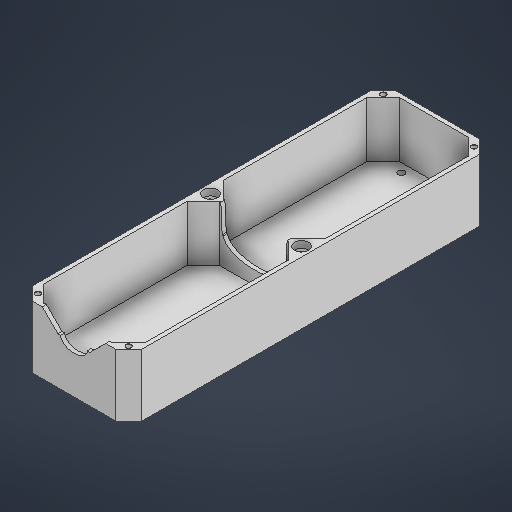
# Autodesk Inventor part: DriverFesting
Saved by Autodesk Inventor 2026.1 (Build 301233000, 233)
## iProperties
Created: 2026-01-13
Part Number: DriverFesting
Material: Generic
Document SubType Name: Modeling
Designer: Brynjar
Density: 1 g/cm^3
Appearance: Default
Author: Brynjar
Autodesk Inventor part; units mm, degrees
ref_plane "YZ Plane" through (0, 0, 0) normal (1, 0, 0) x (0, 1, 0)
ref_plane "XZ Plane" through (0, 0, 0) normal (0, 1, 0) x (-1, 0, 0)
ref_plane "XY Plane" through (0, 0, 0) normal (0, 0, 1) x (1, 0, 0)
sketch "Sketch1" plane through (0, 0, 0) normal (0, 1, 0) x (-1, 0, 0)
  line L0 (-15, -136) -> (-66, -136)
  line L1 (-78, -148) -> (-78, -254)
  line L2 (-66, -266) -> (-15, -266)
  line L3 (-3, -254) -> (-3, -148)
  line L4 (-15, -133) -> (-66, -133)
  line L5 (-78, -121) -> (-78, -15)
  line L6 (-66, -3) -> (-15, -3)
  line L7 (-3, -15) -> (-3, -121)
  line L8 (-78, -136) -> (-78, -133) construction
  line L9 (-9.5147, 0) -> (-71.4853, 0)
  line L10 (-81, -9.5147) -> (-81, -259.4853)
  line L11 (-71.4853, -269) -> (-9.5147, -269)
  line L12 (0, -259.4853) -> (0, -9.5147)
  line L13 (-3, -3) -> (0, -3) construction
  line L14 (-3, -3) -> (-3, 0) construction
  line L15 (-78, -266) -> (-78, -269) construction
  line L16 (-78, -266) -> (-81, -266) construction
  line L17 (-3, -201) -> (-78, -201) construction
  line L18 (-23, -142.5) -> (-58, -142.5) construction
  line L19 (-58, -142.5) -> (-58, -259.5) construction
  line L20 (-58, -259.5) -> (-23, -259.5) construction
  line L21 (-23, -259.5) -> (-23, -142.5) construction
  line L22 (-23, -142.5) -> (-58, -259.5) construction
  line L23 (-58, -142.5) -> (-23, -259.5) construction
  circle A0 centre (-23, -259.5) radius 2.5
  circle A1 centre (-58, -259.5) radius 2.5
  circle A2 centre (-58, -142.5) radius 2.5
  circle A3 centre (-23, -142.5) radius 2.5
  line L24 (-15, -266) -> (-3, -254)
  line L25 (-66, -266) -> (-78, -254)
  line L26 (-3, -148) -> (-15, -136)
  line L27 (-66, -136) -> (-78, -148)
  line L28 (-15, -133) -> (-3, -121)
  line L29 (-66, -133) -> (-78, -121)
  line L30 (-3, -15) -> (-15, -3)
  line L31 (-66, -3) -> (-78, -15)
  line L32 (0, -259.4853) -> (-9.5147, -269)
  line L33 (-81, -259.4853) -> (-71.4853, -269)
  line L34 (-71.4853, 0) -> (-81, -9.5147)
  line L35 (0, -9.5147) -> (-9.5147, 0)
  line L36 (-4.7574, -264.2426) -> (-9, -260) construction
  circle A4 centre (-6.8345, -134.5) radius 2.5
  circle A5 centre (-74.1655, -134.5) radius 2.5
  circle A6 centre (-6.8345, -134.5) radius 6.8345 construction
  circle A7 centre (-74.1655, -134.5) radius 6.8345 construction
  circle A8 centre (-6.8345, -134.5) radius 5.25
  circle A9 centre (-74.1655, -134.5) radius 5.25
  point P0 (0, 0)
  point P1 (-3, -136)
  point P2 (-3, -266)
  point P3 (-3, -133)
  point P4 (-78, -3)
  point P5 (-81, -269)
  point P6 (-81, 0)
  point P7 (0, -269)
  point P8 (-40.5, -201)
  dimension "d0" = 75
  dimension "d1" = 130
  dimension "d2" = 3
  dimension "d3" = 130
  dimension "d4" = 117
  dimension "d5" = 5
  dimension "d6" = 35
  dimension "d27" = 135
  dimension "d28" = 12
  dimension "d42" = 10.5
  dimension "d48" = 6
  constraints: 74 end point, 28 point on line, 15 equal length, 14 perpendicular, 13 parallel, 10 centre point, 8 coincident, 7 midpoint, 6 equal radius, 6 tangent, 4 horizontal, 1 vertical
  measures "d0" distance of point (-3, -266) L15.start
  measures "d1" distance of L15.start L8.start
  measures "d2" distance of L8.start L8.end
  measures "d3" distance of L8.end point (-78, -3)
  measures "d4" distance of L18.end L19.end
  measures "d5" diameter of A0
  measures "d6" distance of L19.end L20.end
  measures "d27" angle of L2 L24
  measures "d28" distance of L2.end point (-3, -266)
  measures "d42" diameter of A8
  measures "d48" distance of L36.start L36.end
extrude "Extrusion1" add sketch "Sketch1" against normal blind 5 contours L26 L3 L24 L2 L25 L1 L27 L0 | L4 L29 L5 L31 L6 L30 L7 L28 | L35 L12 L32 L11 L33 L10 L34 L9 | A8 | A9
extrude "Extrusion2" add sketch "Sketch1" along normal blind 41 contours L35 L12 L32 L11 L33 L10 L34 L9 | A8 | A9
sketch "Sketch2" plane through (13.7574, -3, -133) normal (0, 0, 1) x (1, 0, 0)
  line L0 (26.7426, 13) -> (26.7426, 3) construction
  line L1 (-10.7574, 23.5) -> (3.2426, 23.5) construction
  line L2 (-10.7574, 3) -> (-10.7574, 44) construction
  line L3 (52.2426, 3) -> (1.2426, 3) construction
  ellipse E0 centre (26.7426, 23.5) end of major axis (49.2426, 23.5) minor radius 10.5
  line L4 (26.7426, 23.5) -> (4.2426, 23.5) construction
  line L5 (26.7426, 23.5) -> (26.7426, 13) construction
  line L6 (3.2426, 23.5) -> (2.2426, 44)
  line L7 (3.2426, 23.5) -> (4.2426, 23.5)
  line L8 (1.2426, 44) -> (2.2426, 44)
  line L9 (50.2426, 23.5) -> (51.2426, 44)
  line L10 (50.2426, 23.5) -> (49.2426, 23.5)
  line L11 (52.2426, 44) -> (51.2426, 44)
  line L12 (2.2426, 44) -> (51.2426, 44)
  point P0 (-13.7574, 3)
  point P1 (49.2426, 23.5)
  dimension "d38" = 10
  dimension "d39" = 15
  dimension "d67" = 1
  constraints: 22 end point, 4 horizontal, 4 symmetric about line, 2 midpoint, 2 vertical, 1 parallel, 4 other
  measures "d38" distance of L0.end L0.start
  measures "d39" distance of L1.start L4.end
  measures "d67" distance of L1.end L4.end
extrude "Extrusion3" cut sketch "Sketch2" against normal up to next
sketch "Sketch3" plane through (0, 41, 0) normal (0, 1, 0) x (1, 0, 0)
  circle A0 centre (6.8345, 134.5) radius 5.25 projected
  circle A1 centre (74.1655, 134.5) radius 5.25 projected
  point P0 (0, 0)
extrude "Extrusion4" cut sketch "Sketch3" against normal blind 5
sketch "Sketch5" plane through (0, 41, 0) normal (0, 1, 0) x (1, 0, 0)
  line L0 (0, 9.5147) -> (9.5147, 0) construction
  line L1 (15, 3) -> (3, 15) construction
  line L2 (4.7574, 4.7574) -> (9, 9) construction
  circle A0 centre (6.8787, 6.8787) radius 1.85
  circle A1 centre (6.8787, 6.8787) radius 1.5 construction
  circle A2 centre (6.8787, 6.8787) radius 2.05
  point P0 (0, 0)
  dimension "d53" = 3.7
  dimension "d54" = 3
  dimension "d55" = 4.1
  constraints: 3 centre point, 3 midpoint, 2 coincident, 2 end point
  measures "d53" diameter of A0
  measures "d54" diameter of A1
  measures "d55" diameter of A2
extrude "Extrusion6" cut sketch "Sketch5" against normal blind 6.2 contours A0
extrude "Extrusion7" cut sketch "Sketch5" against normal blind 0.2 contours A0 | A2
sketch "Sketch6" plane through (0, 41, 0) normal (0, 1, 0) x (1, 0, 0)
  line L0 (71.4853, 0) -> (81, 9.5147) construction
  line L1 (78, 15) -> (66, 3) construction
  line L2 (81, 259.4853) -> (71.4853, 269) construction
  line L3 (66, 266) -> (78, 254) construction
  line L4 (9.5147, 269) -> (0, 259.4853) construction
  line L5 (3, 254) -> (15, 266) construction
  line L6 (76.2426, 4.7574) -> (72, 9) construction
  line L7 (76.2426, 264.2426) -> (72, 260) construction
  line L8 (4.7574, 264.2426) -> (9, 260) construction
  point P0 (0, 0)
  point P1 (6.8787, 262.1213)
  point P2 (74.1213, 262.1213)
  point P3 (74.1213, 6.8787)
  constraints: 9 midpoint, 6 end point
pattern_sketch "Sketch Driven Pattern1" of "Extrusion6", "Extrusion7" from (6.8787, 41, -6.8787) copies at (6.8787, 41, -262.1213) at (74.1213, 41, -262.1213) at (74.1213, 41, -6.8787)
sketch "Sketch7" plane through (9.5147, -5, 0) normal (0, 0, 1) x (1, 0, 0)
  ellipse E0 centre (30.9853, 34.5) end of major axis (40.8314, 34.5) minor radius 6.5
  line L0 (30.9853, 34.5) -> (40.8314, 34.5) construction
  line L1 (30.9853, 34.5) -> (30.9853, 41) construction
  line L2 (30.9853, 46) -> (30.9853, 41) construction
  line L3 (5.4853, 5) -> (5.4853, 46) construction
  line L4 (56.4853, 5) -> (56.4853, 46) construction
  line L5 (7.4853, 46) -> (19.1391, 34.5)
  line L6 (19.1391, 34.5) -> (21.1391, 34.5)
  line L7 (54.4853, 46) -> (42.8314, 34.5)
  line L8 (42.8314, 34.5) -> (40.8314, 34.5)
  line L9 (5.4853, 46) -> (7.4853, 46)
  line L10 (56.4853, 46) -> (54.4853, 46)
  line L11 (7.4853, 46) -> (54.4853, 46)
  point P0 (-9.5147, 5)
  dimension "d61" = 6.5
  dimension "d62" = 9.8461
  dimension "d63" = 5
  dimension "d64" = 2
  constraints: 20 end point, 4 equal length, 4 horizontal, 2 vertical, 1 collinear, 1 midpoint, 5 other
  measures "d61" distance of L0.start L1.end
  measures "d62" distance of L0.start L0.end
  measures "d63" distance of L2.start L1.end
  measures "d64" distance of L4.end L7.start
extrude "Extrusion8" cut sketch "Sketch7" against normal up to next
equation "\"d3\" = d1"
body "Solid1"
